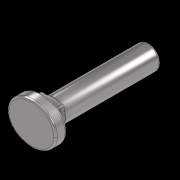
# Autodesk Inventor part: skaterScrew
Saved by Autodesk Inventor 2022.2 (Build 262287010, 287A)
## iProperties
Created: 2022-04-27
Part Number: skaterScrew
Material: Stainless Steel
Document SubType Name: Modeling
Designer: Árni Þór Þorgeirsson
Density: 8 g/cm^3
Appearance: Semi-Polished
Author: Árni Þór Þorgeirsson
Autodesk Inventor part; units mm, degrees
ref_plane "YZ Plane" through (0, 0, 0) normal (1, 0, 0) x (0, 1, 0)
ref_plane "XZ Plane" through (0, 0, 0) normal (0, 1, 0) x (-1, 0, 0)
ref_plane "XY Plane" through (0, 0, 0) normal (0, 0, 1) x (1, 0, 0)
sketch "Sketch1" plane through (0, 0, 0) normal (0, 0, 1) x (1, 0, 0)
  circle A0 centre (0, 0) radius 3.1
  circle A1 centre (0, 0) radius 2.4
  dimension "d0" = 6.2
  dimension "d1" = 4.8
  constraints: 2 centre point, 2 coincident
  measures "d0" diameter of A0
  measures "d1" diameter of A1
extrude "Extrusion1" add sketch "Sketch1" along normal blind 25.5
sketch "Sketch2" plane through (0, 0, 25.5) normal (0, 0, 1) x (1, 0, 0)
  line L0 (-3.175, 3.175) -> (3.175, 3.175)
  line L1 (3.175, 3.175) -> (3.175, -3.175)
  line L2 (3.175, -3.175) -> (-3.175, -3.175)
  line L3 (-3.175, -3.175) -> (-3.175, 3.175)
  circle A0 centre (0, 0) radius 2.4 projected
  line L4 (-3.175, 3.175) -> (3.175, -3.175) construction
  line L5 (3.175, 3.175) -> (-3.175, -3.175) construction
  dimension "d4" = 6.35
  dimension "d5" = 6.35
  constraints: 12 end point, 2 midpoint, 2 parallel, 1 horizontal, 1 perpendicular
  measures "d4" distance of L1.end L2.end
  measures "d5" distance of L0.end L1.end
extrude "Extrusion2" add sketch "Sketch2" along normal blind 2.5 contours L0 L1 L2 L3 | A0
sketch "Sketch3" plane through (0, 0, 28) normal (0, 0, 1) x (1, 0, 0)
  ellipse E0 centre (0, 0) end of major axis (6.4, 0) minor radius 5.45
  dimension "d8" = 5.45
  dimension "d9" = 6.4
  constraints: 1 centre point, 1 coincident, 1 other
extrude "Extrusion3" add sketch "Sketch3" along normal blind 3
fillet "Fillet1" radius 0.5 2 edges at (-6.4, 0, 31) (-6.4, 0, 28)
fillet "Fillet2" radius 0.5 10 edges at (-3.175, 3.175, 26.75) (3.175, 3.175, 26.75) (0, 3.175, 28) (-3.175, 0, 28) (-3.175, -3.175, 26.75) (0, -3.175, 28) (3.175, -3.175, 26.75) (3.175, 0, 28) (-3.1, 0, 25.5) (-3.1, 0, 0)
thread "Thread1" size "M5x0.8" class "6H" standard "ANSI Metric M Profile" full length
body "Solid1"
